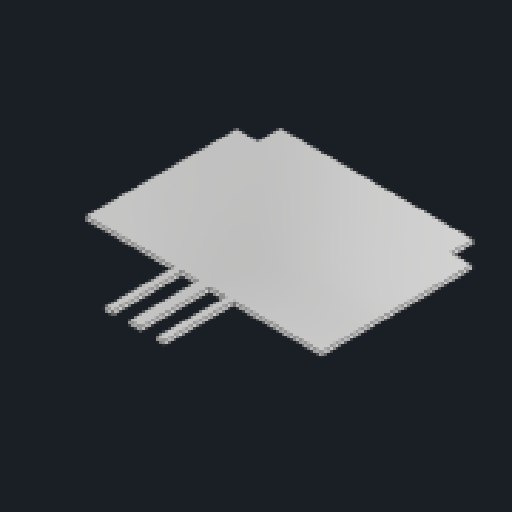
# Autodesk Inventor part: base
Saved by Autodesk Inventor 2023 (Build 270158000, 158)
## iProperties
Created: 2024-04-10
Part Number: base
Material: Aluminum 6061-AHC
Document SubType Name: Modeling
Designer: szymo
Density: 2.7 g/cm^3
Appearance: Aluminum - Dark
Mass: 197.721 g
Surface Area: 516.1 cm^2
Volume: 73.23 cm^3
Author: szymo
Autodesk Inventor part; units mm, degrees
ref_plane "YZ Plane" through (0, 0, 0) normal (1, 0, 0) x (0, 1, 0)
ref_plane "XZ Plane" through (0, 0, 0) normal (0, 1, 0) x (-1, 0, 0)
ref_plane "XY Plane" through (0, 0, 0) normal (0, 0, 1) x (1, 0, 0)
sketch "Sketch2" plane through (0, 0, 0) normal (0, 1, 0) x (-1, 0, 0)
  line L0 (-89, 99) -> (89, 99)
  line L1 (89, 99) -> (89, -99)
  line L2 (89, -99) -> (-89, -99)
  line L3 (-89, -99) -> (-89, 99)
  line L4 (-89, 99) -> (89, -99) construction
  line L5 (89, 99) -> (-89, -99) construction
  line L6 (-89, 99) -> (89, 99)
  line L7 (89, 99) -> (89, -85)
  line L8 (89, -85) -> (-89, -85)
  line L9 (-89, -85) -> (-89, 99)
  line L10 (-4.5, 99) -> (-89, 99)
  line L11 (-89, 99) -> (-89, 46)
  line L12 (-89, 46) -> (-4.5, 46)
  line L13 (-4.5, 46) -> (-4.5, 99)
  line L14 (4.5, 99) -> (89, 99)
  line L15 (89, 99) -> (89, 46)
  line L16 (89, 46) -> (4.5, 46)
  line L17 (4.5, 46) -> (4.5, 99)
  line L18 (22.5, 77.5) -> (22.5, 66.5) projected
  line L19 (16.5, 66.5) -> (16.5, 77.5) projected
  line L20 (-22.5, 66.5) -> (-22.5, 77.5) projected
  line L21 (-16.5, 77.5) -> (-16.5, 66.5) projected
  line L22 (-22.5, 99) -> (-16.5, 99)
  line L23 (-16.5, 99) -> (-16.5, 46)
  line L24 (-16.5, 46) -> (-22.5, 46)
  line L25 (-22.5, 46) -> (-22.5, 99)
  line L26 (16.5, 99) -> (22.5, 99)
  line L27 (22.5, 99) -> (22.5, 46)
  line L28 (22.5, 46) -> (16.5, 46)
  line L29 (16.5, 46) -> (16.5, 99)
  line L30 (-89, 99) -> (89, 99)
  line L31 (89, 99) -> (89, 98)
  line L32 (89, 98) -> (-89, 98)
  line L33 (-89, 98) -> (-89, 99)
  line L34 (89, -85) -> (73, -85)
  line L35 (73, -85) -> (73, -68)
  line L36 (73, -68) -> (89, -68)
  line L37 (89, -68) -> (89, -85)
  line L38 (-89, -85) -> (-73, -85)
  line L39 (-73, -85) -> (-73, -68)
  line L40 (-73, -68) -> (-89, -68)
  line L41 (-89, -68) -> (-89, -85)
  point P0 (0, 0)
  point P1 (4.5, 99)
  point P2 (-4.5, 99)
  point P3 (-89, 46)
  point P4 (89, 46)
  point P5 (4.5, 98)
  point P6 (-4.5, 98)
  point P7 (-16.5, 98)
  point P8 (-22.5, 98)
  point P9 (22.5, 98)
  point P10 (16.5, 98)
  point P11 (73, -85)
  dimension "d8" = 178
  dimension "d9" = 198
  dimension "d10" = 14
  dimension "d11" = 84.5
  dimension "d12" = 53
  dimension "d13" = 84.5
  dimension "d14" = 53
  dimension "d17" = 9
  dimension "d18" = 1
  dimension "d19" = 16
  dimension "d20" = 17
  dimension "d21" = 16
  dimension "d22" = 17
  constraints: 76 end point, 18 parallel, 9 horizontal, 9 perpendicular, 7 point on line, 4 collinear, 2 midpoint, 5 other
  measures "d8" distance of L1.end L2.end
  measures "d9" distance of L0.end L1.end
  measures "d10" distance between parallel lines of L8 L2
  measures "d11" distance of L12.end L11.end
  measures "d12" distance of L0.start L11.end
  measures "d13" distance of L15.end L16.end
  measures "d14" distance of L6.end L15.end
  measures "d17" distance between parallel lines of L13 L17
  measures "d18" distance of L30.end L31.end
  measures "d19" distance of L35.end L36.end
  measures "d20" distance of L34.end L35.end
  measures "d21" distance of L40.end L39.end
  measures "d22" distance of L39.end L38.end
extrude "Extrusion2" add sketch "Sketch2" along normal blind 3 contours L32 L23 L21 L12 L25 L20 | L12 L13 L32 L17 L16 L1 L36 L35 L8 L39 L40 L3 | L32 L27 L18 L16 L29 L19
equation "\"d11\" = d13"
body "Solid2"
